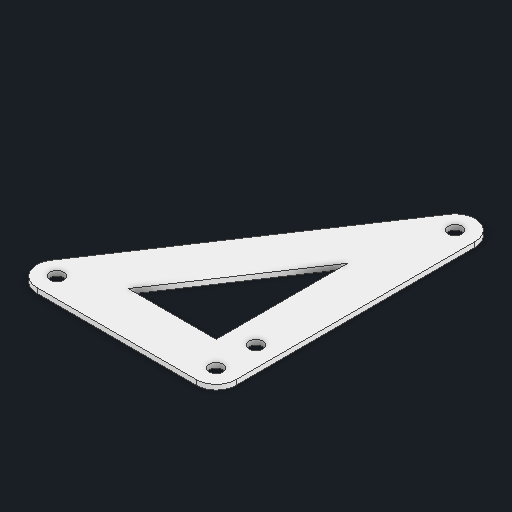
# Autodesk Inventor part: Triangle Gusset
Saved by Autodesk Inventor 2025.1 (Build 291241000, 241)
## iProperties
Created: 2024-12-30
Part Number: Triangle Gusset
Material: Acetal Resin, White
Document SubType Name: Modeling
Designer: Averey Ku
Density: 1.425 g/cm^3
Appearance: Smooth - White
Author: Averey Ku
Autodesk Inventor part; units mm, degrees
ref_plane "YZ Plane" through (0, 0, 0) normal (1, 0, 0) x (0, 1, 0)
ref_plane "XZ Plane" through (0, 0, 0) normal (0, 1, 0) x (-1, 0, 0)
ref_plane "XY Plane" through (0, 0, 0) normal (0, 0, 1) x (1, 0, 0)
sketch "main" plane through (0, 0, 0) normal (0, 0, 1) x (1, 0, 0)
  circle A0 centre (-24.2926, 27.4457) radius 2.1844
  circle A1 centre (-24.2926, -48.7543) radius 2.1844
  circle A2 centre (26.5074, 27.4457) radius 2.1844
  arc A3 (-30.6426, -48.7543) -> (-19.0091, -52.2766) centre (-24.2926, -48.7543) ccw
  arc A4 (31.7909, 23.9234) -> (26.5074, 33.7957) centre (26.5074, 27.4457) ccw
  arc A5 (-24.2926, 33.7957) -> (-30.6426, 27.4457) centre (-24.2926, 27.4457) ccw
  line L0 (-30.6426, -48.7543) -> (-30.6426, 27.4457)
  line L1 (-24.2926, 33.7957) -> (26.5074, 33.7957)
  line L2 (31.7909, 23.9234) -> (-19.0091, -52.2766)
  line L3 (-16.3551, -22.5385) -> (11.6761, 19.5082)
  line L4 (11.6761, 19.5082) -> (-16.3551, 19.5082)
  line L5 (-16.3551, 19.5082) -> (-16.3551, -22.5385)
  circle A6 centre (-24.2926, 14.7457) radius 2.1844
  point P0 (-7.9432, 11.0963)
  dimension "d0" = 12.7
  dimension "d1" = 12.7
  dimension "d2" = 12.7
  dimension "d3" = 14.2875
  dimension "d6" = 4.3688
  dimension "d7" = 76.2
  dimension "d8" = 0
  measures "d0" diameter of A4
  measures "d1" diameter of A5
  measures "d2" diameter of A3
  measures "d3" distance between parallel lines of L2 L3
  measures "d6" diameter of A6
  measures "d7" distance of A0.centre A1.centre
  measures "d8" horizontal distance of A0.centre A1.centre
sketch "Sketch1" plane through (0, 0, 0) normal (0, 1, 0) x (-1, 0, 0)
  circle A0 centre (0, 0) radius 2.1844
  circle A1 centre (0, -76.2) radius 2.1844
  circle A2 centre (50.8, 0) radius 2.1844
  arc A3 (-6.35, -76.2) -> (5.2835, -79.7223) centre (0, -76.2) ccw
  arc A4 (56.0835, -3.5223) -> (50.8, 6.35) centre (50.8, 0) ccw
  arc A5 (0, 6.35) -> (-6.35, 0) centre (0, 0) ccw
  line L0 (-6.35, -76.2) -> (-6.35, 0)
  line L1 (0, 6.35) -> (50.8, 6.35)
  line L2 (56.0835, -3.5223) -> (5.2835, -79.7223)
  line L3 (7.9375, -49.9842) -> (35.9686, -7.9375)
  line L4 (35.9686, -7.9375) -> (7.9375, -7.9375)
  line L5 (7.9375, -7.9375) -> (7.9375, -49.9842)
  circle A6 centre (0, -12.7) radius 2.1844
  constraints: 1 other
extrude "Extrusion1" add sketch "Sketch1" along normal blind 1.5875
body "Solid1"
